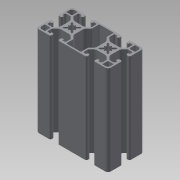
# Autodesk Inventor part: 40-4080-UL
Saved by Autodesk Inventor 2013 (Build 170138000, 138)
## iProperties
Created: 2014-04-23
Part Number: 40-4080-UL
Material: Generic
Document SubType Name: Modeling
Designer: Ross Bowman
Density: 1 g/cm^3
Engineer: Ross Bowman
Catalog Web Link: 8020.net
Vendor: 80/20 Inc.
Company: 80/20 Inc.
Author: Ross Bowman
Keywords: 80/20 , 8020 , T-Slot , Extrusion
Material: 6105-T5 Aluminum
Autodesk Inventor part; units mm, degrees
ref_plane "YZ Plane" through (0, 0, 0) normal (1, 0, 0) x (0, 1, 0)
ref_plane "XZ Plane" through (0, 0, 0) normal (0, 1, 0) x (-1, 0, 0)
ref_plane "XY Plane" through (0, 0, 0) normal (0, 0, 1) x (1, 0, 0)
sketch "Sketch1" plane through (0, 0, 0) normal (0, 0, 1) x (1, 0, 0)
  line L0 (25.1263, -3.712) -> (23.0049, -1.5907)
  line L1 (25.4393, -4.8481) -> (25.1263, -3.712)
  arc A0 (24.8481, -5.4393) -> (25.4393, -4.8481) centre (24.9497, -4.9497) ccw
  line L2 (23.712, -5.1263) -> (24.8481, -5.4393)
  line L3 (21.5907, -3.0049) -> (23.712, -5.1263)
  arc A1 (20.625, -3.3421) -> (21.5907, -3.0049) centre (20, 0) ccw
  line L4 (20.4923, -4.0876) -> (20.625, -3.3421)
  arc A2 (19.5077, -4.0876) -> (20.4923, -4.0876) centre (20, -4) ccw
  line L5 (19.375, -3.3421) -> (19.5077, -4.0876)
  arc A3 (18.4093, -3.0049) -> (19.375, -3.3421) centre (20, 0) ccw
  line L6 (16.288, -5.1263) -> (18.4093, -3.0049)
  line L7 (15.1519, -5.4393) -> (16.288, -5.1263)
  arc A4 (14.5607, -4.8481) -> (15.1519, -5.4393) centre (15.0503, -4.9497) ccw
  line L8 (14.8737, -3.712) -> (14.5607, -4.8481)
  line L9 (16.9951, -1.5907) -> (14.8737, -3.712)
  arc A5 (16.6579, -0.625) -> (16.9951, -1.5907) centre (20, 0) ccw
  line L10 (15.9124, -0.4923) -> (16.6579, -0.625)
  arc A6 (15.9124, 0.4923) -> (15.9124, -0.4923) centre (16, 0) ccw
  line L11 (16.6579, 0.625) -> (15.9124, 0.4923)
  arc A7 (16.9951, 1.5907) -> (16.6579, 0.625) centre (20, 0) ccw
  line L12 (14.8737, 3.712) -> (16.9951, 1.5907)
  line L13 (14.5607, 4.8481) -> (14.8737, 3.712)
  arc A8 (15.1519, 5.4393) -> (14.5607, 4.8481) centre (15.0503, 4.9497) ccw
  line L14 (16.288, 5.1263) -> (15.1519, 5.4393)
  line L15 (18.4093, 3.0049) -> (16.288, 5.1263)
  arc A9 (19.375, 3.3421) -> (18.4093, 3.0049) centre (20, 0) ccw
  line L16 (19.5077, 4.0876) -> (19.375, 3.3421)
  arc A10 (20.4923, 4.0876) -> (19.5077, 4.0876) centre (20, 4) ccw
  line L17 (20.625, 3.3421) -> (20.4923, 4.0876)
  arc A11 (21.5907, 3.0049) -> (20.625, 3.3421) centre (20, 0) ccw
  line L18 (23.712, 5.1263) -> (21.5907, 3.0049)
  line L19 (24.8481, 5.4393) -> (23.712, 5.1263)
  arc A12 (25.4393, 4.8481) -> (24.8481, 5.4393) centre (24.9497, 4.9497) ccw
  line L20 (25.1263, 3.712) -> (25.4393, 4.8481)
  line L21 (23.0049, 1.5907) -> (25.1263, 3.712)
  arc A13 (23.3421, 0.625) -> (23.0049, 1.5907) centre (20, 0) ccw
  line L22 (24.0876, 0.4923) -> (23.3421, 0.625)
  arc A14 (24.0876, -0.4923) -> (24.0876, 0.4923) centre (24, 0) ccw
  line L23 (23.3421, -0.625) -> (24.0876, -0.4923)
  arc A15 (23.0049, -1.5907) -> (23.3421, -0.625) centre (20, 0) ccw
  line L24 (-14.8737, -3.712) -> (-16.9951, -1.5907)
  line L25 (-14.5607, -4.8481) -> (-14.8737, -3.712)
  arc A16 (-15.1519, -5.4393) -> (-14.5607, -4.8481) centre (-15.0503, -4.9497) ccw
  line L26 (-16.288, -5.1263) -> (-15.1519, -5.4393)
  line L27 (-18.4093, -3.0049) -> (-16.288, -5.1263)
  arc A17 (-19.375, -3.3421) -> (-18.4093, -3.0049) centre (-20, 0) ccw
  line L28 (-19.5077, -4.0876) -> (-19.375, -3.3421)
  arc A18 (-20.4923, -4.0876) -> (-19.5077, -4.0876) centre (-20, -4) ccw
  line L29 (-20.625, -3.3421) -> (-20.4923, -4.0876)
  arc A19 (-21.5907, -3.0049) -> (-20.625, -3.3421) centre (-20, 0) ccw
  line L30 (-23.712, -5.1263) -> (-21.5907, -3.0049)
  line L31 (-24.8481, -5.4393) -> (-23.712, -5.1263)
  arc A20 (-25.4393, -4.8481) -> (-24.8481, -5.4393) centre (-24.9497, -4.9497) ccw
  line L32 (-25.1263, -3.712) -> (-25.4393, -4.8481)
  line L33 (-23.0049, -1.5907) -> (-25.1263, -3.712)
  arc A21 (-23.3421, -0.625) -> (-23.0049, -1.5907) centre (-20, 0) ccw
  line L34 (-24.0876, -0.4923) -> (-23.3421, -0.625)
  arc A22 (-24.0876, 0.4923) -> (-24.0876, -0.4923) centre (-24, 0) ccw
  line L35 (-23.3421, 0.625) -> (-24.0876, 0.4923)
  arc A23 (-23.0049, 1.5907) -> (-23.3421, 0.625) centre (-20, 0) ccw
  line L36 (-25.1263, 3.712) -> (-23.0049, 1.5907)
  line L37 (-25.4393, 4.8481) -> (-25.1263, 3.712)
  arc A24 (-24.8481, 5.4393) -> (-25.4393, 4.8481) centre (-24.9497, 4.9497) ccw
  line L38 (-23.712, 5.1263) -> (-24.8481, 5.4393)
  line L39 (-21.5907, 3.0049) -> (-23.712, 5.1263)
  arc A25 (-20.625, 3.3421) -> (-21.5907, 3.0049) centre (-20, 0) ccw
  line L40 (-20.4923, 4.0876) -> (-20.625, 3.3421)
  arc A26 (-19.5077, 4.0876) -> (-20.4923, 4.0876) centre (-20, 4) ccw
  line L41 (-19.375, 3.3421) -> (-19.5077, 4.0876)
  arc A27 (-18.4093, 3.0049) -> (-19.375, 3.3421) centre (-20, 0) ccw
  line L42 (-16.288, 5.1263) -> (-18.4093, 3.0049)
  line L43 (-15.1519, 5.4393) -> (-16.288, 5.1263)
  arc A28 (-14.5607, 4.8481) -> (-15.1519, 5.4393) centre (-15.0503, 4.9497) ccw
  line L44 (-14.8737, 3.712) -> (-14.5607, 4.8481)
  line L45 (-16.9951, 1.5907) -> (-14.8737, 3.712)
  arc A29 (-16.6579, 0.625) -> (-16.9951, 1.5907) centre (-20, 0) ccw
  line L46 (-15.9124, 0.4923) -> (-16.6579, 0.625)
  arc A30 (-15.9124, -0.4923) -> (-15.9124, 0.4923) centre (-16, 0) ccw
  line L47 (-16.6579, -0.625) -> (-15.9124, -0.4923)
  arc A31 (-16.9951, -1.5907) -> (-16.6579, -0.625) centre (-20, 0) ccw
  arc A32 (38.345, 15.545) -> (35.545, 18.345) centre (35.545, 15.545) ccw
  line L48 (38.345, 12.4898) -> (38.345, 15.545)
  arc A33 (37.715, 11.8598) -> (38.345, 12.4898) centre (37.715, 12.4898) ccw
  line L49 (33.1298, 11.8598) -> (37.715, 11.8598)
  arc A34 (31.8598, 13.1298) -> (33.1298, 11.8598) centre (33.1298, 13.1298) ccw
  line L50 (31.8598, 17.715) -> (31.8598, 13.1298)
  arc A35 (32.4898, 18.345) -> (31.8598, 17.715) centre (32.4898, 17.715) ccw
  line L51 (35.545, 18.345) -> (32.4898, 18.345)
  arc A36 (-35.545, 18.345) -> (-38.345, 15.545) centre (-35.545, 15.545) ccw
  line L52 (-32.4898, 18.345) -> (-35.545, 18.345)
  arc A37 (-31.8598, 17.715) -> (-32.4898, 18.345) centre (-32.4898, 17.715) ccw
  line L53 (-31.8598, 13.1298) -> (-31.8598, 17.715)
  arc A38 (-33.1298, 11.8598) -> (-31.8598, 13.1298) centre (-33.1298, 13.1298) ccw
  line L54 (-37.715, 11.8598) -> (-33.1298, 11.8598)
  arc A39 (-38.345, 12.4898) -> (-37.715, 11.8598) centre (-37.715, 12.4898) ccw
  line L55 (-38.345, 15.545) -> (-38.345, 12.4898)
  arc A40 (-38.345, -15.545) -> (-35.545, -18.345) centre (-35.545, -15.545) ccw
  line L56 (-38.345, -12.4898) -> (-38.345, -15.545)
  arc A41 (-37.715, -11.8598) -> (-38.345, -12.4898) centre (-37.715, -12.4898) ccw
  line L57 (-33.1298, -11.8598) -> (-37.715, -11.8598)
  arc A42 (-31.8598, -13.1298) -> (-33.1298, -11.8598) centre (-33.1298, -13.1298) ccw
  line L58 (-31.8598, -17.715) -> (-31.8598, -13.1298)
  arc A43 (-32.4898, -18.345) -> (-31.8598, -17.715) centre (-32.4898, -17.715) ccw
  line L59 (-35.545, -18.345) -> (-32.4898, -18.345)
  arc A44 (8.1402, 17.715) -> (7.5102, 18.345) centre (7.5102, 17.715) ccw
  line L60 (8.1402, 10.8233) -> (8.1402, 17.715)
  arc A45 (8.1402, 10.8233) -> (8.5122, 9.9253) centre (9.4102, 10.8233) ccw
  line L61 (10.9238, 7.5137) -> (8.5122, 9.9253)
  arc A46 (12.315, 4.1549) -> (10.9238, 7.5137) centre (7.565, 4.1549) ccw
  line L62 (12.315, -4.1549) -> (12.315, 4.1549)
  arc A47 (10.9238, -7.5137) -> (12.315, -4.1549) centre (7.565, -4.1549) ccw
  line L63 (8.5122, -9.9253) -> (10.9238, -7.5137)
  arc A48 (8.5122, -9.9253) -> (8.1402, -10.8233) centre (9.4102, -10.8233) ccw
  line L64 (8.1402, -17.715) -> (8.1402, -10.8233)
  arc A49 (7.5102, -18.345) -> (8.1402, -17.715) centre (7.5102, -17.715) ccw
  line L65 (-7.5102, -18.345) -> (7.5102, -18.345)
  arc A50 (-8.1402, -17.715) -> (-7.5102, -18.345) centre (-7.5102, -17.715) ccw
  line L66 (-8.1402, -10.8233) -> (-8.1402, -17.715)
  arc A51 (-8.1402, -10.8233) -> (-8.5122, -9.9253) centre (-9.4102, -10.8233) ccw
  line L67 (-10.9238, -7.5137) -> (-8.5122, -9.9253)
  arc A52 (-12.315, -4.1549) -> (-10.9238, -7.5137) centre (-7.565, -4.1549) ccw
  line L68 (-12.315, 4.1549) -> (-12.315, -4.1549)
  arc A53 (-10.9238, 7.5137) -> (-12.315, 4.1549) centre (-7.565, 4.1549) ccw
  line L69 (-8.5122, 9.9253) -> (-10.9238, 7.5137)
  arc A54 (-8.5122, 9.9253) -> (-8.1402, 10.8233) centre (-9.4102, 10.8233) ccw
  line L70 (-8.1402, 17.715) -> (-8.1402, 10.8233)
  arc A55 (-7.5102, 18.345) -> (-8.1402, 17.715) centre (-7.5102, 17.715) ccw
  line L71 (7.5102, 18.345) -> (-7.5102, 18.345)
  arc A56 (35.545, -18.345) -> (38.345, -15.545) centre (35.545, -15.545) ccw
  line L72 (32.4898, -18.345) -> (35.545, -18.345)
  arc A57 (31.8598, -17.715) -> (32.4898, -18.345) centre (32.4898, -17.715) ccw
  line L73 (31.8598, -13.1298) -> (31.8598, -17.715)
  arc A58 (33.1298, -11.8598) -> (31.8598, -13.1298) centre (33.1298, -13.1298) ccw
  line L74 (37.715, -11.8598) -> (33.1298, -11.8598)
  arc A59 (38.345, -12.4898) -> (37.715, -11.8598) centre (37.715, -12.4898) ccw
  line L75 (38.345, -15.545) -> (38.345, -12.4898)
  arc A60 (-25.569, -20) -> (-24, -18.4848) centre (-25.569, -18.43) ccw
  line L76 (-24, -18.4848) -> (-24, -17.255)
  arc A61 (-24, -17.255) -> (-25.57, -15.685) centre (-25.57, -17.255) ccw
  line L77 (-25.57, -15.685) -> (-26.474, -15.685)
  arc A62 (-26.474, -15.685) -> (-26.855, -16.066) centre (-26.474, -16.066) ccw
  line L78 (-26.855, -16.066) -> (-26.855, -17.119)
  arc A63 (-27.236, -17.5) -> (-26.855, -17.119) centre (-27.236, -17.119) ccw
  line L79 (-27.236, -17.5) -> (-29.015, -17.5)
  arc A64 (-30.285, -16.23) -> (-29.015, -17.5) centre (-29.015, -16.23) ccw
  line L80 (-30.285, -16.23) -> (-30.285, -12.2162)
  arc A65 (-30.0243, -11.5869) -> (-30.285, -12.2162) centre (-29.395, -12.2162) ccw
  line L81 (-30.0243, -11.5869) -> (-27.5137, -9.0762)
  arc A66 (-24.1549, -7.685) -> (-27.5137, -9.0762) centre (-24.1549, -12.435) ccw
  line L82 (-24.1549, -7.685) -> (-15.8451, -7.685)
  arc A67 (-12.4863, -9.0762) -> (-15.8451, -7.685) centre (-15.8451, -12.435) ccw
  line L83 (-12.4863, -9.0762) -> (-9.9757, -11.5869)
  arc A68 (-9.715, -12.2162) -> (-9.9757, -11.5869) centre (-10.605, -12.2162) ccw
  line L84 (-9.715, -12.2162) -> (-9.715, -16.23)
  arc A69 (-10.985, -17.5) -> (-9.715, -16.23) centre (-10.985, -16.23) ccw
  line L85 (-10.985, -17.5) -> (-12.764, -17.5)
  arc A70 (-13.145, -17.119) -> (-12.764, -17.5) centre (-12.764, -17.119) ccw
  line L86 (-13.145, -17.119) -> (-13.145, -16.066)
  arc A71 (-13.145, -16.066) -> (-13.526, -15.685) centre (-13.526, -16.066) ccw
  line L87 (-13.526, -15.685) -> (-14.43, -15.685)
  arc A72 (-14.43, -15.685) -> (-16, -17.255) centre (-14.43, -17.255) ccw
  line L88 (-16, -17.255) -> (-16, -18.4848)
  arc A73 (-16, -18.4848) -> (-14.431, -20) centre (-14.431, -18.43) ccw
  line L89 (-14.431, -20) -> (14.43, -20)
  arc A74 (14.43, -20) -> (16, -18.43) centre (14.43, -18.43) ccw
  line L90 (16, -18.43) -> (16, -17.255)
  arc A75 (16, -17.255) -> (14.43, -15.685) centre (14.43, -17.255) ccw
  line L91 (14.43, -15.685) -> (13.526, -15.685)
  arc A76 (13.526, -15.685) -> (13.145, -16.066) centre (13.526, -16.066) ccw
  line L92 (13.145, -16.066) -> (13.145, -17.119)
  arc A77 (12.764, -17.5) -> (13.145, -17.119) centre (12.764, -17.119) ccw
  line L93 (12.764, -17.5) -> (10.985, -17.5)
  arc A78 (9.715, -16.23) -> (10.985, -17.5) centre (10.985, -16.23) ccw
  line L94 (9.715, -16.23) -> (9.715, -12.2162)
  arc A79 (9.9757, -11.5869) -> (9.715, -12.2162) centre (10.605, -12.2162) ccw
  line L95 (9.9757, -11.5869) -> (12.4863, -9.0762)
  arc A80 (15.8451, -7.685) -> (12.4863, -9.0762) centre (15.8451, -12.435) ccw
  line L96 (15.8451, -7.685) -> (24.1549, -7.685)
  arc A81 (27.5137, -9.0762) -> (24.1549, -7.685) centre (24.1549, -12.435) ccw
  line L97 (27.5137, -9.0762) -> (30.0243, -11.5869)
  arc A82 (30.285, -12.2162) -> (30.0243, -11.5869) centre (29.395, -12.2162) ccw
  line L98 (30.285, -12.2162) -> (30.285, -16.23)
  arc A83 (29.015, -17.5) -> (30.285, -16.23) centre (29.015, -16.23) ccw
  line L99 (29.015, -17.5) -> (27.236, -17.5)
  arc A84 (26.855, -17.119) -> (27.236, -17.5) centre (27.236, -17.119) ccw
  line L100 (26.855, -17.119) -> (26.855, -16.066)
  arc A85 (26.855, -16.066) -> (26.474, -15.685) centre (26.474, -16.066) ccw
  line L101 (26.474, -15.685) -> (25.57, -15.685)
  arc A86 (25.57, -15.685) -> (24, -17.255) centre (25.57, -17.255) ccw
  line L102 (24, -17.255) -> (24, -18.43)
  arc A87 (24, -18.43) -> (25.57, -20) centre (25.57, -18.43) ccw
  line L103 (25.57, -20) -> (36.83, -20)
  arc A88 (36.83, -20) -> (40, -16.83) centre (36.83, -16.83) ccw
  line L104 (40, -16.83) -> (40, -5.57)
  arc A89 (40, -5.57) -> (38.43, -4) centre (38.43, -5.57) ccw
  line L105 (38.43, -4) -> (37.255, -4)
  arc A90 (37.255, -4) -> (35.685, -5.57) centre (37.255, -5.57) ccw
  line L106 (35.685, -5.57) -> (35.685, -6.474)
  arc A91 (35.685, -6.474) -> (36.066, -6.855) centre (36.066, -6.474) ccw
  line L107 (36.066, -6.855) -> (37.119, -6.855)
  arc A92 (37.5, -7.236) -> (37.119, -6.855) centre (37.119, -7.236) ccw
  line L108 (37.5, -7.236) -> (37.5, -9.015)
  arc A93 (36.23, -10.285) -> (37.5, -9.015) centre (36.23, -9.015) ccw
  line L109 (36.23, -10.285) -> (32.2162, -10.285)
  arc A94 (31.5869, -10.0243) -> (32.2162, -10.285) centre (32.2162, -9.395) ccw
  line L110 (31.5869, -10.0243) -> (29.0762, -7.5137)
  arc A95 (27.685, -4.1549) -> (29.0762, -7.5137) centre (32.435, -4.1549) ccw
  line L111 (27.685, -4.1549) -> (27.685, 4.1549)
  arc A96 (29.0762, 7.5137) -> (27.685, 4.1549) centre (32.435, 4.1549) ccw
  line L112 (29.0762, 7.5137) -> (31.5869, 10.0243)
  arc A97 (32.2162, 10.285) -> (31.5869, 10.0243) centre (32.2162, 9.395) ccw
  line L113 (32.2162, 10.285) -> (36.23, 10.285)
  arc A98 (37.5, 9.015) -> (36.23, 10.285) centre (36.23, 9.015) ccw
  line L114 (37.5, 9.015) -> (37.5, 7.236)
  arc A99 (37.119, 6.855) -> (37.5, 7.236) centre (37.119, 7.236) ccw
  line L115 (37.119, 6.855) -> (36.066, 6.855)
  arc A100 (36.066, 6.855) -> (35.685, 6.474) centre (36.066, 6.474) ccw
  line L116 (35.685, 6.474) -> (35.685, 5.57)
  arc A101 (35.685, 5.57) -> (37.255, 4) centre (37.255, 5.57) ccw
  line L117 (37.255, 4) -> (38.43, 4)
  arc A102 (38.43, 4) -> (40, 5.57) centre (38.43, 5.57) ccw
  line L118 (40, 5.57) -> (40, 16.83)
  arc A103 (40, 16.83) -> (36.83, 20) centre (36.83, 16.83) ccw
  line L119 (36.83, 20) -> (25.57, 20)
  arc A104 (25.57, 20) -> (24, 18.43) centre (25.57, 18.43) ccw
  line L120 (24, 18.43) -> (24, 17.255)
  arc A105 (24, 17.255) -> (25.57, 15.685) centre (25.57, 17.255) ccw
  line L121 (25.57, 15.685) -> (26.474, 15.685)
  arc A106 (26.474, 15.685) -> (26.855, 16.066) centre (26.474, 16.066) ccw
  line L122 (26.855, 16.066) -> (26.855, 17.119)
  arc A107 (27.236, 17.5) -> (26.855, 17.119) centre (27.236, 17.119) ccw
  line L123 (27.236, 17.5) -> (29.015, 17.5)
  arc A108 (30.285, 16.23) -> (29.015, 17.5) centre (29.015, 16.23) ccw
  line L124 (30.285, 16.23) -> (30.285, 12.2162)
  arc A109 (30.0243, 11.5869) -> (30.285, 12.2162) centre (29.395, 12.2162) ccw
  line L125 (30.0243, 11.5869) -> (27.5137, 9.0762)
  arc A110 (24.1549, 7.685) -> (27.5137, 9.0762) centre (24.1549, 12.435) ccw
  line L126 (24.1549, 7.685) -> (15.8451, 7.685)
  arc A111 (12.4863, 9.0762) -> (15.8451, 7.685) centre (15.8451, 12.435) ccw
  line L127 (12.4863, 9.0762) -> (9.9757, 11.5869)
  arc A112 (9.715, 12.2162) -> (9.9757, 11.5869) centre (10.605, 12.2162) ccw
  line L128 (9.715, 12.2162) -> (9.715, 16.23)
  arc A113 (10.985, 17.5) -> (9.715, 16.23) centre (10.985, 16.23) ccw
  line L129 (10.985, 17.5) -> (12.764, 17.5)
  arc A114 (13.145, 17.119) -> (12.764, 17.5) centre (12.764, 17.119) ccw
  line L130 (13.145, 17.119) -> (13.145, 16.066)
  arc A115 (13.145, 16.066) -> (13.526, 15.685) centre (13.526, 16.066) ccw
  line L131 (13.526, 15.685) -> (14.43, 15.685)
  arc A116 (14.43, 15.685) -> (16, 17.255) centre (14.43, 17.255) ccw
  line L132 (16, 17.255) -> (16, 18.43)
  arc A117 (16, 18.43) -> (14.43, 20) centre (14.43, 18.43) ccw
  line L133 (14.43, 20) -> (-14.43, 20)
  arc A118 (-14.43, 20) -> (-16, 18.43) centre (-14.43, 18.43) ccw
  line L134 (-16, 18.43) -> (-16, 17.255)
  arc A119 (-16, 17.255) -> (-14.43, 15.685) centre (-14.43, 17.255) ccw
  line L135 (-14.43, 15.685) -> (-13.526, 15.685)
  arc A120 (-13.526, 15.685) -> (-13.145, 16.066) centre (-13.526, 16.066) ccw
  line L136 (-13.145, 16.066) -> (-13.145, 17.119)
  arc A121 (-12.764, 17.5) -> (-13.145, 17.119) centre (-12.764, 17.119) ccw
  line L137 (-12.764, 17.5) -> (-10.985, 17.5)
  arc A122 (-9.715, 16.23) -> (-10.985, 17.5) centre (-10.985, 16.23) ccw
  line L138 (-9.715, 16.23) -> (-9.715, 12.2162)
  arc A123 (-9.9757, 11.5869) -> (-9.715, 12.2162) centre (-10.605, 12.2162) ccw
  line L139 (-9.9757, 11.5869) -> (-12.4863, 9.0762)
  arc A124 (-15.8451, 7.685) -> (-12.4863, 9.0762) centre (-15.8451, 12.435) ccw
  line L140 (-15.8451, 7.685) -> (-24.1549, 7.685)
  arc A125 (-27.5137, 9.0762) -> (-24.1549, 7.685) centre (-24.1549, 12.435) ccw
  line L141 (-27.5137, 9.0762) -> (-30.0243, 11.5869)
  arc A126 (-30.285, 12.2162) -> (-30.0243, 11.5869) centre (-29.395, 12.2162) ccw
  line L142 (-30.285, 12.2162) -> (-30.285, 16.23)
  arc A127 (-29.015, 17.5) -> (-30.285, 16.23) centre (-29.015, 16.23) ccw
  line L143 (-29.015, 17.5) -> (-27.236, 17.5)
  arc A128 (-26.855, 17.119) -> (-27.236, 17.5) centre (-27.236, 17.119) ccw
  line L144 (-26.855, 17.119) -> (-26.855, 16.066)
  arc A129 (-26.855, 16.066) -> (-26.474, 15.685) centre (-26.474, 16.066) ccw
  line L145 (-26.474, 15.685) -> (-25.57, 15.685)
  arc A130 (-25.57, 15.685) -> (-24, 17.255) centre (-25.57, 17.255) ccw
  line L146 (-24, 17.255) -> (-24, 18.43)
  arc A131 (-24, 18.43) -> (-25.57, 20) centre (-25.57, 18.43) ccw
  line L147 (-25.57, 20) -> (-36.83, 20)
  arc A132 (-36.83, 20) -> (-40, 16.83) centre (-36.83, 16.83) ccw
  line L148 (-40, 16.83) -> (-40, 5.57)
  arc A133 (-40, 5.57) -> (-38.43, 4) centre (-38.43, 5.57) ccw
  line L149 (-38.43, 4) -> (-37.255, 4)
  arc A134 (-37.255, 4) -> (-35.685, 5.57) centre (-37.255, 5.57) ccw
  line L150 (-35.685, 5.57) -> (-35.685, 6.474)
  arc A135 (-35.685, 6.474) -> (-36.066, 6.855) centre (-36.066, 6.474) ccw
  line L151 (-36.066, 6.855) -> (-37.119, 6.855)
  arc A136 (-37.5, 7.236) -> (-37.119, 6.855) centre (-37.119, 7.236) ccw
  line L152 (-37.5, 7.236) -> (-37.5, 9.015)
  arc A137 (-36.23, 10.285) -> (-37.5, 9.015) centre (-36.23, 9.015) ccw
  line L153 (-36.23, 10.285) -> (-32.2162, 10.285)
  arc A138 (-31.5869, 10.0243) -> (-32.2162, 10.285) centre (-32.2162, 9.395) ccw
  line L154 (-31.5869, 10.0243) -> (-29.0762, 7.5137)
  arc A139 (-27.685, 4.1549) -> (-29.0762, 7.5137) centre (-32.435, 4.1549) ccw
  line L155 (-27.685, 4.1549) -> (-27.685, -4.1549)
  arc A140 (-29.0762, -7.5137) -> (-27.685, -4.1549) centre (-32.435, -4.1549) ccw
  line L156 (-29.0762, -7.5137) -> (-31.5869, -10.0243)
  arc A141 (-32.2162, -10.285) -> (-31.5869, -10.0243) centre (-32.2162, -9.395) ccw
  line L157 (-32.2162, -10.285) -> (-36.23, -10.285)
  arc A142 (-37.5, -9.015) -> (-36.23, -10.285) centre (-36.23, -9.015) ccw
  line L158 (-37.5, -9.015) -> (-37.5, -7.236)
  arc A143 (-37.119, -6.855) -> (-37.5, -7.236) centre (-37.119, -7.236) ccw
  line L159 (-37.119, -6.855) -> (-36.066, -6.855)
  arc A144 (-36.066, -6.855) -> (-35.685, -6.474) centre (-36.066, -6.474) ccw
  line L160 (-35.685, -6.474) -> (-35.685, -5.57)
  arc A145 (-35.685, -5.57) -> (-37.255, -4) centre (-37.255, -5.57) ccw
  line L161 (-37.255, -4) -> (-38.43, -4)
  arc A146 (-38.43, -4) -> (-40, -5.57) centre (-38.43, -5.57) ccw
  line L162 (-40, -5.57) -> (-40, -16.83)
  arc A147 (-40, -16.83) -> (-36.83, -20) centre (-36.83, -16.83) ccw
  line L163 (-36.83, -20) -> (-25.569, -20)
  point P0 (0, 0)
  constraints: 328 end point, 296 point on circle, 148 centre point
extrude "Extrusion1" add sketch "Sketch1" against normal blind 100
body "Solid1"
